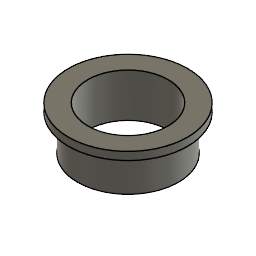
Shaft-Spacer-For-Magnet-Distance (Autodesk Fusion 360 design; units mm, degrees)
Autodesk Fusion 360 part; units mm, degrees
sketch "Sketch1" plane through (0, 0, 0) normal (0, 1, 0) x (1, 0, 0)
  circle A0 centre (0, 0) radius 5.05
  circle A1 centre (0, 0) radius 6.35
  dimension "d1" = 10.1
  dimension "d2" = 12.7
  constraint coincident A0.centre A1.centre
  constraint concentric A0 A1
  measures "d1" diameter of A0
  measures "d2" diameter of A1
extrude "Extrude1" add sketch "Sketch1" along normal blind 5.5
sketch "Sketch2" plane through (0, 5.5, 0) normal (0, 1, 0) x (-1, 0, 0)
  circle A0 centre (0, 0) radius 5.05
  circle A1 centre (0, 0) radius 6.35
  circle A2 centre (0, 0) radius 7.5
  constraint concentric A0 A2
extrude "Extrude2" add sketch "Sketch2" against normal blind 1 contours A2
equation "d2 = 10.1 mm + 2.6 mm"
